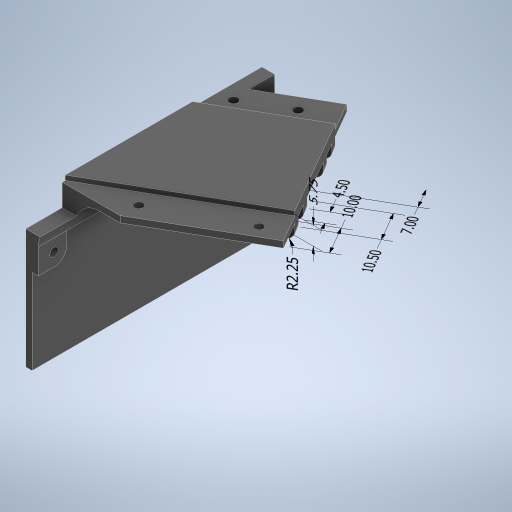
# Autodesk Inventor part: flame_side_right
Saved by Autodesk Inventor 2024.1 (Build 281209000, 209)
## iProperties
Created: 2025-03-06
Part Number: flame_side_right
Material: 一般
Document SubType Name: Modeling
Designer: hibik
Density: 1 g/cm^3
Appearance: 既定
Author: hibik
Autodesk Inventor part; units mm, degrees
ref_plane "YZ Plane" through (0, 0, 0) normal (1, 0, 0) x (0, 1, 0)
ref_plane "XZ Plane" through (0, 0, 0) normal (0, 1, 0) x (-1, 0, 0)
ref_plane "XY Plane" through (0, 0, 0) normal (0, 0, 1) x (1, 0, 0)
sketch "スケッチ1" plane through (0, 0, 0) normal (0, 1, 0) x (-1, 0, 0)
  line L0 (0, 0) -> (-75, 129.9038)
  line L1 (0, 0) -> (9.1573, 5.287) construction
  line L2 (-46.25, 80.1073) -> (0, 106.8098)
  line L3 (-28.75, 49.7965) -> (0, 66.3953)
  line L4 (-37.5, 64.9519) -> (-18.3005, 76.0367) construction
  line L5 (25.9887, 0) -> (-91.8315, 0) projected
  line L6 (0, 0) -> (0, 106.8098)
  line L7 (-51.25, 88.7676) -> (0, 118.3568)
  line L8 (0, 118.3568) -> (0, 106.8098)
  line L9 (-23.75, 41.1362) -> (0, 54.8483)
  dimension "d0" = 150
  dimension "d1" = 60
  dimension "d2" = 57.5
  dimension "d5" = 10
  constraints: 18 end point, 6 point on line, 4 perpendicular, 2 vertical, 1 midpoint, 1 parallel, 2 other
  measures "d0" distance from line of L0.end L1
  measures "d1" angle of L0 L5
  measures "d2" distance between parallel lines of L1 L3
  measures "d5" distance between parallel lines of L3 L9
extrude "押し出し1" add sketch "スケッチ1" along normal blind 1.5 contours L0 L2 L6 L3
extrude "押し出し2" add sketch "スケッチ1" against normal blind 2 contours L0 L3 L6 L9 | L0 L2 L6 L3 | L0 L7 L8 L2
sketch "スケッチ2" plane through (0, 1.5, 66.3953) normal (-1, 0, 0) x (0, 0, 1)
  line L0 (-22.0385, -1.5) -> (52.9615, -1.5)
  line L1 (52.9615, -1.5) -> (52.9615, -46.5)
  line L2 (52.9615, -46.5) -> (-22.0385, -46.5)
  line L3 (-22.0385, -46.5) -> (-22.0385, -1.5)
  line L4 (40.4145, -1.5) -> (51.9615, -1.5) projected
  line L5 (-22.0385, -11.5) -> (52.9615, -11.5)
  line L6 (51.9615, -3.5) -> (-11.547, -3.5) projected
  line L7 (51.9615, -1.5) -> (51.9615, -3.5) projected
  point P0 (-66.3953, -1.5)
  point P1 (20.2073, -3.5)
  point P2 (15.4615, -11.5)
  dimension "d8" = 75
  dimension "d9" = 35
  dimension "d12" = 10
  dimension "d23" = 1
  constraints: 10 end point, 2 midpoint, 2 parallel, 2 perpendicular, 2 point on line, 1 collinear, 1 horizontal
  measures "d8" distance of L0.start L0.end
  measures "d9" distance between parallel lines of L2 L5
  measures "d12" distance between parallel lines of L0 L5
  measures "d23" distance between parallel lines of L7 L1
extrude "押し出し3" add sketch "スケッチ2" against normal blind 2
sketch "スケッチ3" plane through (2, 1.5, 66.3953) normal (1, 0, 0) x (0, 0, -1)
  circle A0 centre (-47.9615, -15.5) radius 4
  circle A1 centre (17.0385, -15.5) radius 4
  line L0 (-52.9615, -46.5) -> (22.0385, -46.5) projected
  line L1 (-52.9615, -11.5) -> (22.0385, -11.5)
  line L2 (22.0385, -46.5) -> (22.0385, -1.5) projected
  line L3 (-51.9615, -11.5) -> (-51.9615, -18.5112) construction
  line L4 (-52.9615, -11.5) -> (-43.9615, -11.5)
  line L5 (-43.9615, -11.5) -> (-43.9615, -19.5)
  line L6 (-43.9615, -19.5) -> (-52.9615, -19.5)
  line L7 (-52.9615, -19.5) -> (-52.9615, -11.5)
  line L8 (22.0385, -11.5) -> (13.0385, -11.5)
  line L9 (13.0385, -11.5) -> (13.0385, -19.5)
  line L10 (13.0385, -19.5) -> (22.0385, -19.5)
  line L11 (22.0385, -19.5) -> (22.0385, -11.5)
  line L12 (22.0385, -1.5) -> (0, -1.5) projected
  line L13 (0, 0) -> (-40.4145, 0) projected
  line L14 (-40.4145, -1.5) -> (0, -1.5) projected
  line L15 (-40.4145, -1.5) -> (-40.4145, 0) projected
  line L16 (0, -1.5) -> (0, 0) projected
  line L17 (-40.4145, -1.5) -> (0, -1.5)
  line L18 (-52.9615, -1.5) -> (-52.9615, -46.5) projected
  line L19 (-40.4145, -1.5) -> (-52.9615, -1.5) projected
  point P0 (66.3953, -1.5)
  point P1 (13.0385, -15.5)
  point P2 (17.0385, -19.5)
  point P3 (22.0385, -19.5)
  point P4 (13.0385, -11.5)
  point P5 (-47.9615, -19.5)
  point P6 (-43.9615, -15.5)
  point P7 (-47.9615, -11.5)
  dimension "d13" = 8
  dimension "d14" = 35
  dimension "d15" = 65
  dimension "d24" = 1
  constraints: 22 end point, 7 tangent, 4 horizontal, 4 parallel, 2 centre point, 2 perpendicular, 2 point on line, 1 collinear, 1 equal radius, 1 vertical
  measures "d13" diameter of A0
  measures "d14" distance between parallel lines of L0 L1
  measures "d15" distance of A1.centre A0.centre
  measures "d24" distance between parallel lines of L18 L3
extrude "押し出し4" add sketch "スケッチ3" along normal blind 2 contours A0 | A0 L1 L5 | A0 L6 L7 L1 | L1 L18 L19 L14 L12 L2 | L1 A1 L9 | L1 L2 L10 A1 | A1
sketch "スケッチ4" plane through (4, 1.5, 66.3953) normal (1, 0, 0) x (0, 0, -1)
  arc A0 (-47.9615, -19.5) -> (-43.9615, -15.5) centre (-47.9615, -15.5) ccw projected
  arc A1 (13.0385, -15.5) -> (17.0385, -19.5) centre (17.0385, -15.5) ccw projected
  circle A2 centre (-47.9615, -15.5) radius 1.35
  circle A3 centre (17.0385, -15.5) radius 1.35
  point P0 (66.3953, -1.5)
  dimension "d19" = 2.7
  dimension "d20" = 2.7
  constraints: 2 centre point, 2 coincident
  measures "d19" diameter of A2
  measures "d20" diameter of A3
extrude "押し出し5" cut sketch "スケッチ4" against normal through all
sketch "スケッチ5" plane through (0, -2, 0) normal (0, -1, 0) x (1, 0, 0)
  line L0 (31.6173, 108.7628) -> (-5, 108.7628) construction
  line L1 (51.25, 88.7676) -> (4, 116.0474) projected
  line L2 (0, 44.3568) -> (0, 119.3568) projected
  line L3 (18.3494, 107.7628) -> (0, 107.7628)
  line L4 (4, 116.0474) -> (4, 119.3568) projected
  line L5 (0, 119.3568) -> (4, 119.3568) projected
  point P0 (0, 0)
  point P1 (0, 106.8098)
  dimension "d25" = 1
  constraints: 2 end point, 2 point on line, 1 parallel
  measures "d25" distance between parallel lines of L0 L3
extrude "押し出し6" cut sketch "スケッチ5" along normal mid plane 10
fillet "フィレット1" radius 8 1 edges at (4, -2, 80.1508)
sketch "スケッチ6" plane through (0, 0, 0) normal (0, 1, 0) x (1, 0, 0)
  circle A0 centre (17.5897, -50.4663) radius 1.6 construction
  circle A1 centre (4.5994, -57.9663) radius 1.6 construction
  circle A2 centre (43.3666, -88.7131) radius 1.6 construction
  circle A3 centre (18.4391, -101.9375) radius 1.6 construction
  circle A4 centre (17.5897, -50.4663) radius 1.35
  circle A5 centre (4.5994, -57.9663) radius 1.35
  circle A6 centre (18.4391, -101.9375) radius 1.35
  circle A7 centre (43.3666, -88.7131) radius 1.35
  point P0 (0, 0)
  dimension "d29" = 2.7
  constraints: 4 centre point, 4 coincident, 3 equal radius
  measures "d29" diameter of A4
extrude "押し出し7" cut sketch "スケッチ6" against normal through all
ref_plane "作業平面2" through (3.75, 0, 72.8905) normal (-0.5, 0, -0.8660254) x (-0.8660254, 0, 0.5)
ref_plane "作業平面1" through (8.75, 0, 81.5507) normal (-0.5, 0, -0.8660254) x (-0.8660254, 0, 0.5)
sketch "スケッチ7" plane through (3.75, 0, 72.8905) normal (-0.5, 0, -0.8660254) x (-0.8660254, 0, 0.5)
  circle A0 centre (-30.9476, -4.25) radius 2.25
  circle A1 centre (-30.9476, -4.25) radius 1
  line L0 (-33.1976, -2) -> (4.7927, -2) projected
  line L1 (-33.1976, 0) -> (-33.1976, -2) projected
  line L2 (-33.1976, -2) -> (-33.1976, -4.25)
  line L3 (-28.6976, -4.25) -> (-28.6976, -2)
  point P0 (-30.9476, -2)
  dimension "d33" = 2
  dimension "d34" = 4.5
  constraints: 4 end point, 3 tangent, 2 centre point, 2 point on circle, 1 coincident, 1 parallel, 1 point on line, 1 vertical
  measures "d33" diameter of A1
  measures "d34" diameter of A0
extrude "押し出し8" add sketch "スケッチ7" against normal blind 3
sketch "スケッチ8" plane through (0, 0, 66.3953) normal (-0.5, 0, -0.8660254) x (-0.8660254, 0, 0.5)
  arc A0 (-33.1976, -4.25) -> (-28.6976, -4.25) centre (-30.9476, -4.25) ccw projected
  circle A1 centre (-30.9476, -4.25) radius 1 projected
  line L0 (-28.6976, -4.25) -> (-28.6976, -2) projected
  line L1 (-33.1976, -2) -> (-28.6976, -2) projected
  line L2 (-33.1976, -2) -> (-33.1976, -4.25) projected
  point P0 (-33.1976, 0)
extrude "押し出し9" add sketch "スケッチ8" against normal blind 3
mirror "ミラー1" about plane through (8.75, 0, 81.5507) normal (-0.5, 0, -0.8660254) of "押し出し9", "押し出し8"
